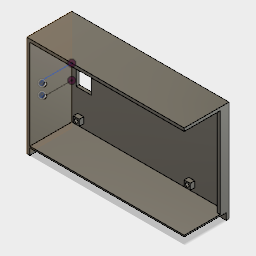
Feather Nephel Housing v9 (Autodesk Fusion 360 design; units mm, degrees)
Autodesk Fusion 360 part; units mm, degrees
sketch "Sketch1" plane through (0, 0, 0) normal (0, 1, 0) x (1, 0, 0)
  line L0 (0, 0) -> (95, 0)
  line L1 (0, 0) -> (-5, 0)
  line L2 (-5, 0) -> (100, 0)
  line L3 (100, 0) -> (100, -2)
  line L4 (100, -2) -> (-5, -2)
  line L5 (-5, -2) -> (-5, 0)
  dimension "d1" = 95
  dimension "d2" = 5
  dimension "d3" = 105
  dimension "d4" = 2
  measures "d1" distance of L0.start L0.end
  measures "d2" distance of L0.start L1.end
  measures "d3" distance of L1.end L2.end
  measures "d4" distance of L1.end L4.end
extrude "Extrude1" add sketch "Sketch1" along normal blind 65
sketch "Sketch2" plane through (0, 0, 2) normal (0, 0, 1) x (1, 0, 0)
  line L0 (-5, 0) -> (100, 0)
  line L1 (100, 0) -> (100, 65)
  line L2 (100, 65) -> (-5, 65)
  line L3 (-5, 65) -> (-5, 0)
  line L4 (-5, 0) -> (5, 0)
  line L5 (5, 0) -> (5, 30)
  line L6 (10, 35) -> (0, 35)
  line L7 (0, 35) -> (0, 25)
  line L8 (0, 25) -> (10, 25)
  line L9 (10, 25) -> (10, 35)
  line L10 (10, 35) -> (0, 25) construction
  line L11 (0, 35) -> (10, 25) construction
  point P0 (5, 30)
  dimension "d7" = 10
  dimension "d8" = 10
  measures "d7" distance of L7.end L8.end
  measures "d8" distance of L6.end L7.end
extrude "Extrude2" cut sketch "Sketch2" against normal blind 2 contours L6 L7 L8 L9
sketch "Sketch3" plane through (0, 0, 2) normal (0, 0, 1) x (1, 0, 0)
  line L0 (0, 35) -> (10, 35)
  line L1 (10, 35) -> (10, 25)
  line L2 (10, 25) -> (0, 25)
  line L3 (0, 25) -> (0, 35)
  line L4 (-5, 0) -> (100, 0)
  line L5 (100, 0) -> (100, 65)
  line L6 (100, 65) -> (-5, 65)
  line L7 (-5, 65) -> (-5, 0)
  line L8 (-5, 65) -> (-3, 65)
  line L9 (-3, 65) -> (-3, 0)
  line L10 (-3, 0) -> (-5, 0)
  line L11 (-5, 0) -> (-5, 65)
  line L12 (0, 0) -> (3, 0)
  line L13 (3, 0) -> (3, 8)
  line L14 (5, 6) -> (1, 6)
  line L15 (1, 6) -> (1, 10)
  line L16 (1, 10) -> (5, 10)
  line L17 (5, 10) -> (5, 6)
  line L18 (5, 6) -> (1, 10) construction
  line L19 (1, 6) -> (5, 10) construction
  point P0 (3, 8)
  dimension "d11" = 65
  dimension "d12" = 2
  dimension "d13" = 3
  dimension "d14" = 8
  dimension "d15" = 4
  dimension "d16" = 4
  measures "d11" distance of L6.end L4.start
  measures "d12" distance of L6.end L8.end
  measures "d13" distance of L12.start L12.end
  measures "d14" distance of L12.end P0
  measures "d15" distance of L15.end L16.end
  measures "d16" distance of L14.end L15.end
extrude "Extrude3" add sketch "Sketch3" along normal blind 3 contours L14 L15 L16 L17
sketch "Sketch4" plane through (0, 0, 2) normal (0, 0, 1) x (1, 0, 0)
  line L0 (5, 10) -> (5, 6)
  line L1 (5, 6) -> (1, 6)
  line L2 (1, 6) -> (1, 10)
  line L3 (1, 10) -> (5, 10)
  line L4 (0, 35) -> (10, 35)
  line L5 (10, 35) -> (10, 25)
  line L6 (10, 25) -> (0, 25)
  line L7 (0, 25) -> (0, 35)
  line L8 (-5, 0) -> (100, 0)
  line L9 (100, 0) -> (100, 65)
  line L10 (100, 65) -> (-5, 65)
  line L11 (-5, 65) -> (-5, 0)
  line L12 (0, 0) -> (3, 0)
  line L13 (3, 0) -> (3, 57)
  line L14 (5, 55) -> (1, 55)
  line L15 (1, 55) -> (1, 59)
  line L16 (1, 59) -> (5, 59)
  line L17 (5, 59) -> (5, 55)
  line L18 (5, 55) -> (1, 59) construction
  line L19 (1, 55) -> (5, 59) construction
  point P0 (3, 57)
  dimension "d19" = 3
  dimension "d20" = 57
  measures "d19" distance of L12.start L12.end
  measures "d20" distance of L12.end P0
extrude "Extrude4" add sketch "Sketch4" along normal blind 3 contours L14 L15 L16 L17
sketch "Sketch5" plane through (0, 0, 2) normal (0, 0, 1) x (1, 0, 0)
  line L0 (5, 59) -> (5, 55)
  line L1 (5, 55) -> (1, 55)
  line L2 (1, 55) -> (1, 59)
  line L3 (1, 59) -> (5, 59)
  line L4 (5, 10) -> (5, 6)
  line L5 (5, 6) -> (1, 6)
  line L6 (1, 6) -> (1, 10)
  line L7 (1, 10) -> (5, 10)
  line L8 (0, 35) -> (10, 35)
  line L9 (10, 35) -> (10, 25)
  line L10 (10, 25) -> (0, 25)
  line L11 (0, 25) -> (0, 35)
  line L12 (-5, 0) -> (100, 0)
  line L13 (100, 0) -> (100, 65)
  line L14 (100, 65) -> (-5, 65)
  line L15 (-5, 65) -> (-5, 0)
  line L16 (0, 0) -> (77, 0)
  line L17 (77, 0) -> (77, 8)
  line L18 (79, 10) -> (75, 10)
  line L19 (75, 10) -> (75, 6)
  line L20 (75, 6) -> (79, 6)
  line L21 (79, 6) -> (79, 10)
  line L22 (79, 10) -> (75, 6) construction
  line L23 (75, 10) -> (79, 6) construction
  point P0 (77, 8)
  dimension "d23" = 77
  dimension "d24" = 8
  dimension "d25" = 4
  dimension "d26" = 4
  measures "d23" distance of L16.start L16.end
  measures "d24" distance of L16.end P0
  measures "d25" distance of L19.end L20.end
  measures "d26" distance of L18.end L19.end
extrude "Extrude5" add sketch "Sketch5" along normal blind 3 contours L18 L19 L20 L21
sketch "Sketch6" plane through (0, 0, 2) normal (0, 0, 1) x (1, 0, 0)
  line L0 (79, 6) -> (75, 6)
  line L1 (75, 6) -> (75, 10)
  line L2 (75, 10) -> (79, 10)
  line L3 (79, 10) -> (79, 6)
  line L4 (5, 59) -> (5, 55)
  line L5 (5, 55) -> (1, 55)
  line L6 (1, 55) -> (1, 59)
  line L7 (1, 59) -> (5, 59)
  line L8 (5, 10) -> (5, 6)
  line L9 (5, 6) -> (1, 6)
  line L10 (1, 6) -> (1, 10)
  line L11 (1, 10) -> (5, 10)
  line L12 (0, 35) -> (10, 35)
  line L13 (10, 35) -> (10, 25)
  line L14 (10, 25) -> (0, 25)
  line L15 (0, 25) -> (0, 35)
  line L16 (-5, 0) -> (100, 0)
  line L17 (100, 0) -> (100, 65)
  line L18 (100, 65) -> (-5, 65)
  line L19 (-5, 65) -> (-5, 0)
  line L20 (0, 0) -> (77, 0)
  line L21 (77, 0) -> (77, 57)
  line L22 (79, 55) -> (75, 55)
  line L23 (75, 55) -> (75, 59)
  line L24 (75, 59) -> (79, 59)
  line L25 (79, 59) -> (79, 55)
  line L26 (79, 55) -> (75, 59) construction
  line L27 (75, 55) -> (79, 59) construction
  point P0 (77, 57)
  dimension "d29" = 77
  dimension "d30" = 57
  dimension "d31" = 4
  dimension "d32" = 4
  measures "d29" distance of L20.start L20.end
  measures "d30" distance of L20.end P0
  measures "d31" distance of L22.end L23.end
  measures "d32" distance of L23.end L24.end
extrude "Extrude6" add sketch "Sketch6" along normal blind 3 contours L22 L23 L24 L25
sketch "Sketch7" plane through (0, 0, 5) normal (0, 0, 1) x (1, 0, 0)
  line L0 (5, 59) -> (1, 59)
  line L1 (1, 59) -> (1, 55)
  line L2 (1, 55) -> (5, 55)
  line L3 (5, 55) -> (5, 59)
  line L4 (1, 59) -> (3, 57)
  circle A0 centre (3, 57) radius 1
  dimension "d35" = 2
  measures "d35" diameter of A0
extrude "Extrude7" add sketch "Sketch7" along normal blind 2 contours A0
sketch "Sketch8" plane through (0, 0, 5) normal (0, 0, 1) x (1, 0, 0)
  line L0 (5, 10) -> (1, 10)
  line L1 (1, 10) -> (1, 6)
  line L2 (1, 6) -> (5, 6)
  line L3 (5, 6) -> (5, 10)
  line L4 (1, 6) -> (3, 8)
  circle A0 centre (3, 8) radius 1
  dimension "d38" = 2
  measures "d38" diameter of A0
extrude "Extrude8" add sketch "Sketch8" along normal blind 2 contours A0
sketch "Sketch9" plane through (0, 0, 5) normal (0, 0, 1) x (1, 0, 0)
  line L0 (79, 59) -> (75, 59)
  line L1 (75, 59) -> (75, 55)
  line L2 (75, 55) -> (79, 55)
  line L3 (79, 55) -> (79, 59)
  line L4 (75, 55) -> (77, 55)
  line L5 (77, 55) -> (77, 57)
  circle A0 centre (77, 57) radius 1
  dimension "d41" = 2
  measures "d41" diameter of A0
extrude "Extrude9" add sketch "Sketch9" along normal blind 2 contours A0
sketch "Sketch10" plane through (0, 0, 5) normal (0, 0, 1) x (1, 0, 0)
  line L0 (79, 6) -> (79, 10)
  line L1 (79, 10) -> (75, 10)
  line L2 (75, 10) -> (75, 6)
  line L3 (75, 6) -> (79, 6)
  line L4 (75, 6) -> (77, 6)
  line L5 (77, 6) -> (77, 8)
  circle A0 centre (77, 8) radius 1
extrude "Extrude10" add sketch "Sketch10" along normal blind 2 contours A0
sketch "Sketch11" plane through (0, 0, 2) normal (0, 0, 1) x (1, 0, 0)
  line L0 (79, 59) -> (79, 55)
  line L1 (79, 55) -> (75, 55)
  line L2 (75, 55) -> (75, 59)
  line L3 (75, 59) -> (79, 59)
  line L4 (79, 6) -> (75, 6)
  line L5 (75, 6) -> (75, 10)
  line L6 (75, 10) -> (79, 10)
  line L7 (79, 10) -> (79, 6)
  line L8 (5, 59) -> (5, 55)
  line L9 (5, 55) -> (1, 55)
  line L10 (1, 55) -> (1, 59)
  line L11 (1, 59) -> (5, 59)
  line L12 (5, 10) -> (5, 6)
  line L13 (5, 6) -> (1, 6)
  line L14 (1, 6) -> (1, 10)
  line L15 (1, 10) -> (5, 10)
  line L16 (0, 35) -> (10, 35)
  line L17 (10, 35) -> (10, 25)
  line L18 (10, 25) -> (0, 25)
  line L19 (0, 25) -> (0, 35)
  line L20 (-5, 0) -> (100, 0)
  line L21 (100, 0) -> (100, 65)
  line L22 (100, 65) -> (-5, 65)
  line L23 (-5, 65) -> (-5, 0)
  line L24 (-5, 0) -> (-3, 0)
  line L25 (-3, 0) -> (-3, 65)
  line L26 (-3, 65) -> (-5, 65)
  line L27 (-5, 65) -> (-5, 0)
  dimension "d46" = 65
  dimension "d47" = 2
  measures "d46" distance of L20.start L22.end
  measures "d47" distance of L20.start L24.end
extrude "Extrude11" add sketch "Sketch11" along normal blind 28 contours L20 L22 L23 L24 L25 L26 L27
sketch "Sketch12" plane through (0, 0, 2) normal (0, 0, 1) x (1, 0, 0)
  line L0 (-3, 65) -> (-3, 0)
  line L1 (-3, 0) -> (100, 0)
  line L2 (100, 0) -> (100, 65)
  line L3 (100, 65) -> (-3, 65)
  line L4 (79, 59) -> (79, 55)
  line L5 (79, 55) -> (75, 55)
  line L6 (75, 55) -> (75, 59)
  line L7 (75, 59) -> (79, 59)
  line L8 (79, 6) -> (75, 6)
  line L9 (75, 6) -> (75, 10)
  line L10 (75, 10) -> (79, 10)
  line L11 (79, 10) -> (79, 6)
  line L12 (5, 59) -> (5, 55)
  line L13 (5, 55) -> (1, 55)
  line L14 (1, 55) -> (1, 59)
  line L15 (1, 59) -> (5, 59)
  line L16 (5, 10) -> (5, 6)
  line L17 (5, 6) -> (1, 6)
  line L18 (1, 6) -> (1, 10)
  line L19 (1, 10) -> (5, 10)
  line L20 (0, 35) -> (10, 35)
  line L21 (10, 35) -> (10, 25)
  line L22 (10, 25) -> (0, 25)
  line L23 (0, 25) -> (0, 35)
  line L24 (100, 65) -> (-3, 65)
  line L25 (-3, 65) -> (-3, 63)
  line L26 (-3, 63) -> (100, 63)
  line L27 (100, 63) -> (100, 65)
  dimension "d50" = 2
  measures "d50" distance of L2.end L26.end
extrude "Extrude12" add sketch "Sketch12" along normal blind 28 contours L0 L2 L3 L24 L25 L26 L27
move_face "OffsetFaces3" offset 2.5 1 faces at (30.6667, 0, 0.6667)
sketch "Sketch19" plane through (0, 0, 0) normal (0, 0, -1) x (-1, 0, 0)
  line L0 (-10, 35) -> (0, 35)
  line L1 (0, 35) -> (0, 25)
  line L2 (0, 25) -> (-10, 25)
  line L3 (-10, 25) -> (-10, 35)
  line L4 (-100, -2.5) -> (5, -2.5)
  line L5 (5, -2.5) -> (5, 65)
  line L6 (5, 65) -> (-100, 65)
  line L7 (-100, 65) -> (-100, -2.5)
  line L8 (5, -2.5) -> (-2, -2.5)
  line L9 (-2, -2.5) -> (-2, 0)
  circle A0 centre (-2, 0) radius 1.3
  dimension "d83" = 2.6
  measures "d83" diameter of A0
extrude "Extrude19" cut sketch "Sketch19" against normal blind 2 contours A0
sketch "Sketch20" plane through (0, 0, 0) normal (0, 0, -1) x (-1, 0, 0)
  circle A0 centre (-2, 0) radius 1.3
  line L0 (-10, 35) -> (0, 35)
  line L1 (0, 35) -> (0, 25)
  line L2 (0, 25) -> (-10, 25)
  line L3 (-10, 25) -> (-10, 35)
  line L4 (-100, -2.5) -> (5, -2.5)
  line L5 (5, -2.5) -> (5, 65)
  line L6 (5, 65) -> (-100, 65)
  line L7 (-100, 65) -> (-100, -2.5)
  line L8 (5, -2.5) -> (-8, -2.5)
  line L9 (-8, -2.5) -> (-8, 0)
  circle A1 centre (-8, 0) radius 1.3
  dimension "d86" = 2.6
  measures "d86" diameter of A1
extrude "Extrude20" cut sketch "Sketch20" against normal blind 2 contours A1
sketch "Sketch21" plane through (0, 0, 2) normal (0, 0, 1) x (1, 0, 0)
  circle A0 centre (8, 0) radius 1.3
  circle A1 centre (2, 0) radius 1.3
  line L0 (0, 35) -> (10, 35)
  line L1 (10, 35) -> (10, 25)
  line L2 (10, 25) -> (0, 25)
  line L3 (0, 25) -> (0, 35)
  line L4 (5, 10) -> (5, 6)
  line L5 (5, 6) -> (1, 6)
  line L6 (1, 6) -> (1, 10)
  line L7 (1, 10) -> (5, 10)
  line L8 (5, 59) -> (5, 55)
  line L9 (5, 55) -> (1, 55)
  line L10 (1, 55) -> (1, 59)
  line L11 (1, 59) -> (5, 59)
  line L12 (79, 6) -> (75, 6)
  line L13 (75, 6) -> (75, 10)
  line L14 (75, 10) -> (79, 10)
  line L15 (79, 10) -> (79, 6)
  line L16 (79, 59) -> (79, 55)
  line L17 (79, 55) -> (75, 55)
  line L18 (75, 55) -> (75, 59)
  line L19 (75, 59) -> (79, 59)
  line L20 (100, 63) -> (-3, 63)
  line L21 (-3, 63) -> (-3, -2.5)
  line L22 (-3, -2.5) -> (100, -2.5)
  line L23 (100, -2.5) -> (100, 63)
  line L24 (-3, -2.5) -> (-3, 2)
  line L25 (-3, 2) -> (100, 2)
  line L26 (100, 2) -> (100, 3)
  line L27 (100, 3) -> (-3, 3)
  line L28 (-3, 3) -> (-3, 2)
  dimension "d89" = 103
  dimension "d90" = 1
  measures "d89" distance of L24.end L25.end
  measures "d90" distance of L24.end L27.end
extrude "Extrude21" add sketch "Sketch21" along normal blind 28 contours L21 L23 L25 L26 L27 L28
sketch "Sketch22" plane through (0, 0, 2) normal (0, 0, 1) x (1, 0, 0)
  line L0 (-3, 3) -> (100, 3)
  line L1 (100, 3) -> (100, 63)
  line L2 (100, 63) -> (-3, 63)
  line L3 (-3, 63) -> (-3, 3)
  line L4 (0, 35) -> (10, 35)
  line L5 (10, 35) -> (10, 25)
  line L6 (10, 25) -> (0, 25)
  line L7 (0, 25) -> (0, 35)
  line L8 (5, 10) -> (5, 6)
  line L9 (5, 6) -> (1, 6)
  line L10 (1, 6) -> (1, 10)
  line L11 (1, 10) -> (5, 10)
  line L12 (5, 59) -> (5, 55)
  line L13 (5, 55) -> (1, 55)
  line L14 (1, 55) -> (1, 59)
  line L15 (1, 59) -> (5, 59)
  line L16 (79, 6) -> (75, 6)
  line L17 (75, 6) -> (75, 10)
  line L18 (75, 10) -> (79, 10)
  line L19 (79, 10) -> (79, 6)
  line L20 (79, 59) -> (79, 55)
  line L21 (79, 55) -> (75, 55)
  line L22 (75, 55) -> (75, 59)
  line L23 (75, 59) -> (79, 59)
  line L24 (100, 63) -> (98, 63)
  line L25 (98, 63) -> (98, 3)
  line L26 (98, 3) -> (100, 3)
  line L27 (100, 3) -> (100, 63)
  dimension "d93" = 60
  dimension "d94" = 2
  measures "d93" distance of L1.end L0.end
  measures "d94" distance of L1.end L24.end
extrude "Extrude22" add sketch "Sketch22" along normal blind 4 contours L0 L1 L2 L24 L25 L26 L27
sketch "Sketch23" plane through (0, 0, 0) normal (0, 0, -1) x (-1, 0, 0)
  circle A0 centre (-8, 0) radius 1.3
  circle A1 centre (-2, 0) radius 1.3
  line L0 (-10, 35) -> (0, 35)
  line L1 (0, 35) -> (0, 25)
  line L2 (0, 25) -> (-10, 25)
  line L3 (-10, 25) -> (-10, 35)
  line L4 (-100, -2.5) -> (5, -2.5)
  line L5 (5, -2.5) -> (5, 65)
  line L6 (5, 65) -> (-100, 65)
  line L7 (-100, 65) -> (-100, -2.5)
  line L8 (0, 35) -> (5, 35)
  line L9 (0, 25) -> (5, 25)
  circle A2 centre (-77, 57) radius 2.2
  dimension "d114" = 4.4
  measures "d114" diameter of A2
sketch "Sketch24" plane through (-5, 0, 0) normal (-1, 0, 0) x (0, 0, 1)
  line L0 (0, -2.5) -> (30, -2.5)
  line L1 (30, -2.5) -> (30, 65)
  line L2 (30, 65) -> (0, 65)
  line L3 (0, 65) -> (0, -2.5)
  line L4 (0, 35) -> (20, 35)
  line L5 (20, 35) -> (20, 33.5)
  circle A0 centre (20, 33.5) radius 1.3
  point P0 (0, 35)
  dimension "d97" = 20
  dimension "d98" = 1.5
  dimension "d99" = 2.6
  measures "d97" distance of P0 L4.end
  measures "d98" distance of L4.end L5.end
  measures "d99" diameter of A0
extrude "Extrude23" cut sketch "Sketch24" against normal blind 2 contours A0
sketch "Sketch25" plane through (-5, 0, 0) normal (-1, 0, 0) x (0, 0, 1)
  circle A0 centre (20, 33.5) radius 1.3
  line L0 (0, -2.5) -> (30, -2.5)
  line L1 (30, -2.5) -> (30, 65)
  line L2 (30, 65) -> (0, 65)
  line L3 (0, 65) -> (0, -2.5)
  line L4 (0, 25) -> (20, 25)
  line L5 (20, 25) -> (20, 26.5)
  circle A1 centre (20, 26.5) radius 1.3
  point P0 (0, 25)
  dimension "d102" = 1.5
  dimension "d103" = 2.6
  measures "d102" distance of L4.end L5.end
  measures "d103" diameter of A1
extrude "Extrude24" cut sketch "Sketch25" against normal blind 2 contours A1
extrude "Extrude25" cut 1 faces at (76.6438, 7.7394, 7) along direction (0, 0, -1) blind 7
extrude "Extrude26" cut 1 faces at (2.6504, 8.3043, 7) along direction (0, 0, -1) blind 7
extrude "Extrude27" cut 1 faces at (3.2444, 57.4232, 7) along direction (0, 0, -1) blind 7
extrude "Extrude28" cut 1 faces at (77.3296, 56.9503, 7) along direction (0, 0, -1) blind 7
extrude "Extrude29" cut sketch "Sketch23" against normal blind 1 contours A2
sketch "Sketch26" plane through (0, 0, 0) normal (0, 0, -1) x (-1, 0, 0)
  circle A0 centre (-77, 57) radius 2.2
  circle A1 centre (-3, 57) radius 1
  circle A2 centre (-3, 8) radius 1
  circle A3 centre (-77, 8) radius 1
  circle A4 centre (-8, 0) radius 1.3
  circle A5 centre (-2, 0) radius 1.3
  line L0 (-10, 35) -> (0, 35)
  line L1 (0, 35) -> (0, 25)
  line L2 (0, 25) -> (-10, 25)
  line L3 (-10, 25) -> (-10, 35)
  line L4 (-100, -2.5) -> (5, -2.5)
  line L5 (5, -2.5) -> (5, 65)
  line L6 (5, 65) -> (-100, 65)
  line L7 (-100, 65) -> (-100, -2.5)
  circle A6 centre (-77, 8) radius 2.2
  dimension "d117" = 4.4
  measures "d117" diameter of A6
extrude "Extrude30" cut sketch "Sketch26" against normal blind 1 contours A6
sketch "Sketch27" plane through (0, 0, 0) normal (0, 0, -1) x (-1, 0, 0)
  circle A0 centre (-77, 8) radius 2.2
  circle A1 centre (-77, 57) radius 2.2
  circle A2 centre (-3, 57) radius 1
  circle A3 centre (-3, 8) radius 1
  circle A4 centre (-8, 0) radius 1.3
  circle A5 centre (-2, 0) radius 1.3
  line L0 (-10, 35) -> (0, 35)
  line L1 (0, 35) -> (0, 25)
  line L2 (0, 25) -> (-10, 25)
  line L3 (-10, 25) -> (-10, 35)
  line L4 (-100, -2.5) -> (5, -2.5)
  line L5 (5, -2.5) -> (5, 65)
  line L6 (5, 65) -> (-100, 65)
  line L7 (-100, 65) -> (-100, -2.5)
  circle A6 centre (-3, 57) radius 2.2
  dimension "d120" = 4.4
  measures "d120" diameter of A6
extrude "Extrude31" cut sketch "Sketch27" against normal blind 1 contours A6
sketch "Sketch28" plane through (0, 0, 0) normal (0, 0, -1) x (-1, 0, 0)
  circle A0 centre (-3, 57) radius 2.2
  circle A1 centre (-77, 8) radius 2.2
  circle A2 centre (-77, 57) radius 2.2
  circle A3 centre (-3, 8) radius 1
  circle A4 centre (-8, 0) radius 1.3
  circle A5 centre (-2, 0) radius 1.3
  line L0 (-10, 35) -> (0, 35)
  line L1 (0, 35) -> (0, 25)
  line L2 (0, 25) -> (-10, 25)
  line L3 (-10, 25) -> (-10, 35)
  line L4 (-100, -2.5) -> (5, -2.5)
  line L5 (5, -2.5) -> (5, 65)
  line L6 (5, 65) -> (-100, 65)
  line L7 (-100, 65) -> (-100, -2.5)
  circle A6 centre (-3, 8) radius 2.2
  dimension "d123" = 4.4
  measures "d123" diameter of A6
extrude "Extrude32" cut sketch "Sketch28" against normal blind 1 contours A6
move_face "OffsetFaces4" offset -0.2 1 faces at (3.9988, 8.0498, 2.3333)
move_face "OffsetFaces5" offset -0.2 1 faces at (77.0249, 7.0003, 2.3333)
move_face "OffsetFaces6" offset -0.2 1 faces at (76.0785, 57.3884, 2.3333)
move_face "OffsetFaces7" offset -0.2 1 faces at (2.0603, 56.658, 2.3333)
